Autodesk Inventor part; units mm, degrees
(part 2 of 4)
  line L489 (-4.322, 37.579) -> (-4.3544, 37.6135) construction
  line L490 (-4.3544, 37.6135) -> (-4.3855, 37.6466) construction
  line L491 (-4.3855, 37.6466) -> (-4.4003, 37.6527) construction
  line L492 (-4.4003, 37.6527) -> (-4.4094, 37.6363) construction
  line L493 (-4.4094, 37.6363) -> (-4.4207, 37.616) construction
  line L494 (-4.4207, 37.616) -> (-4.4319, 37.5271) construction
  line L495 (-4.4319, 37.5271) -> (-4.4272, 37.4953) construction
  line L496 (-4.4272, 37.4953) -> (-4.4241, 37.4748) construction
  line L497 (-4.4241, 37.4748) -> (-4.3492, 37.509) construction
  line L498 (-4.3492, 37.509) -> (-4.3297, 37.5398) construction
  spline S99 degree 3 poles (-4.2878, 37.7736) (-4.285, 37.7935) (-4.2987, 37.8243) (-4.3182, 37.842) (-4.353, 37.8735) (-4.3543, 37.8731) (-4.372, 37.8267) (-4.4023, 37.747) (-4.3954, 37.7255) (-4.3415, 37.7317) (-4.3084, 37.7355) (-4.2914, 37.7488) (-4.2878, 37.7736) knots 0 0 0 0 1 1 1 2 2 2 3 3 3 4 4 4 4
  line L499 (-4.2878, 37.7736) -> (-4.285, 37.7935) construction
  line L500 (-4.285, 37.7935) -> (-4.2987, 37.8243) construction
  line L501 (-4.2987, 37.8243) -> (-4.3182, 37.842) construction
  line L502 (-4.3182, 37.842) -> (-4.353, 37.8735) construction
  line L503 (-4.353, 37.8735) -> (-4.3543, 37.8731) construction
  line L504 (-4.3543, 37.8731) -> (-4.372, 37.8267) construction
  line L505 (-4.372, 37.8267) -> (-4.4023, 37.747) construction
  line L506 (-4.4023, 37.747) -> (-4.3954, 37.7255) construction
  line L507 (-4.3954, 37.7255) -> (-4.3415, 37.7317) construction
  line L508 (-4.3415, 37.7317) -> (-4.3084, 37.7355) construction
  line L509 (-4.3084, 37.7355) -> (-4.2914, 37.7488) construction
  line L510 (-4.2914, 37.7488) -> (-4.2878, 37.7736) construction
  spline S100 degree 3 poles (-4.2238, 37.9809) (-4.2021, 38.0154) (-4.229, 38.0724) (-4.267, 38.0724) (-4.3025, 38.0724) (-4.3297, 37.9751) (-4.2996, 37.956) (-4.2687, 37.9365) (-4.2474, 37.9435) (-4.2238, 37.9809) knots 0 0 0 0 1 1 1 2 2 2 3 3 3 3
  line L511 (-4.2238, 37.9809) -> (-4.2021, 38.0154) construction
  line L512 (-4.2021, 38.0154) -> (-4.229, 38.0724) construction
  line L513 (-4.229, 38.0724) -> (-4.267, 38.0724) construction
  line L514 (-4.267, 38.0724) -> (-4.3025, 38.0724) construction
  line L515 (-4.3025, 38.0724) -> (-4.3297, 37.9751) construction
  line L516 (-4.3297, 37.9751) -> (-4.2996, 37.956) construction
  line L517 (-4.2996, 37.956) -> (-4.2687, 37.9365) construction
  line L518 (-4.2687, 37.9365) -> (-4.2474, 37.9435) construction
  line L519 (-4.2474, 37.9435) -> (-4.2238, 37.9809) construction
  spline S101 degree 3 poles (-4.1426, 38.1788) (-4.1247, 38.2004) (-4.1246, 38.2154) (-4.1421, 38.2537) knots 0 0 0 0 1 1 1 1
  line L520 (-4.1426, 38.1788) -> (-4.1247, 38.2004) construction
  line L521 (-4.1247, 38.2004) -> (-4.1246, 38.2154) construction
  line L522 (-4.1246, 38.2154) -> (-4.1421, 38.2537) construction
  line L523 (-4.1421, 38.2537) -> (-4.1639, 38.3016)
  line L524 (-4.1639, 38.3016) -> (-4.1976, 38.26)
  spline S102 degree 3 poles (-4.1976, 38.26) (-4.2413, 38.206) (-4.2416, 38.1518) (-4.1982, 38.1518) (-4.1799, 38.1518) (-4.155, 38.164) (-4.1426, 38.1788) knots 3 3 3 3 4 4 4 5 5 5 5
  line L525 (-4.1976, 38.26) -> (-4.2413, 38.206) construction
  line L526 (-4.2413, 38.206) -> (-4.2416, 38.1518) construction
  line L527 (-4.2416, 38.1518) -> (-4.1982, 38.1518) construction
  line L528 (-4.1982, 38.1518) -> (-4.1799, 38.1518) construction
  line L529 (-4.1799, 38.1518) -> (-4.155, 38.164) construction
  line L530 (-4.155, 38.164) -> (-4.1426, 38.1788) construction
  spline S103 degree 3 poles (-4.038, 38.3715) (-4.0155, 38.3985) (-4.0284, 38.4693) (-4.0557, 38.4693) (-4.0805, 38.4693) (-4.1299, 38.3849) (-4.1171, 38.3643) (-4.1009, 38.338) (-4.0628, 38.3415) (-4.038, 38.3715) knots 0 0 0 0 1 1 1 2 2 2 3 3 3 3
  line L531 (-4.038, 38.3715) -> (-4.0155, 38.3985) construction
  line L532 (-4.0155, 38.3985) -> (-4.0284, 38.4693) construction
  line L533 (-4.0284, 38.4693) -> (-4.0557, 38.4693) construction
  line L534 (-4.0557, 38.4693) -> (-4.0805, 38.4693) construction
  line L535 (-4.0805, 38.4693) -> (-4.1299, 38.3849) construction
  line L536 (-4.1299, 38.3849) -> (-4.1171, 38.3643) construction
  line L537 (-4.1171, 38.3643) -> (-4.1009, 38.338) construction
  line L538 (-4.1009, 38.338) -> (-4.0628, 38.3415) construction
  line L539 (-4.0628, 38.3415) -> (-4.038, 38.3715) construction
  spline S104 degree 3 poles (-3.8872, 38.5577) (-3.8725, 38.5815) (-3.8939, 38.6457) (-3.9165, 38.6457) (-3.9358, 38.6457) (-4.0004, 38.5752) (-4.0014, 38.5531) knots 0 0 0 0 1 1 1 2 2 2 2
  line L540 (-3.8872, 38.5577) -> (-3.8725, 38.5815) construction
  line L541 (-3.8725, 38.5815) -> (-3.8939, 38.6457) construction
  line L542 (-3.8939, 38.6457) -> (-3.9165, 38.6457) construction
  line L543 (-3.9165, 38.6457) -> (-3.9358, 38.6457) construction
  line L544 (-3.9358, 38.6457) -> (-4.0004, 38.5752) construction
  line L545 (-4.0004, 38.5752) -> (-4.0014, 38.5531) construction
  spline S105 degree 3 poles (-4.0014, 38.5531) (-4.0023, 38.5331) (-3.8999, 38.5372) (-3.8872, 38.5577) knots 2 2 2 2 3 3 3 3
  line L546 (-4.0014, 38.5531) -> (-4.0023, 38.5331) construction
  line L547 (-4.0023, 38.5331) -> (-3.8999, 38.5372) construction
  line L548 (-3.8999, 38.5372) -> (-3.8872, 38.5577) construction
  spline S106 degree 3 poles (-3.7405, 38.7393) (-3.7371, 38.7569) (-3.7393, 38.7839) (-3.7452, 38.7995) knots 0 0 0 0 1 1 1 1
  line L549 (-3.7405, 38.7393) -> (-3.7371, 38.7569) construction
  line L550 (-3.7371, 38.7569) -> (-3.7393, 38.7839) construction
  line L551 (-3.7393, 38.7839) -> (-3.7452, 38.7995) construction
  spline S107 degree 3 poles (-3.7452, 38.7995) (-3.7543, 38.8232) (-3.7644, 38.8197) (-3.8078, 38.7781) knots 1 1 1 1 2 2 2 2
  line L552 (-3.7452, 38.7995) -> (-3.7543, 38.8232) construction
  line L553 (-3.7543, 38.8232) -> (-3.7644, 38.8197) construction
  line L554 (-3.7644, 38.8197) -> (-3.8078, 38.7781) construction
  spline S108 degree 3 poles (-3.8078, 38.7781) (-3.8363, 38.7508) (-3.8552, 38.7213) (-3.8497, 38.7126) knots 2 2 2 2 3 3 3 3
  line L555 (-3.8078, 38.7781) -> (-3.8363, 38.7508) construction
  line L556 (-3.8363, 38.7508) -> (-3.8552, 38.7213) construction
  line L557 (-3.8552, 38.7213) -> (-3.8497, 38.7126) construction
  spline S109 degree 3 poles (-3.8497, 38.7126) (-3.8323, 38.6844) (-3.7469, 38.7053) (-3.7405, 38.7393) knots 3 3 3 3 4 4 4 4
  line L558 (-3.8497, 38.7126) -> (-3.8323, 38.6844) construction
  line L559 (-3.8323, 38.6844) -> (-3.7469, 38.7053) construction
  line L560 (-3.7469, 38.7053) -> (-3.7405, 38.7393) construction
  spline S110 degree 3 poles (-3.5972, 38.8708) (-3.5719, 38.8912) (-3.5629, 38.9122) (-3.5706, 38.9325) (-3.5861, 38.9727) (-3.595, 38.9713) (-3.658, 38.9194) (-3.7025, 38.8828) (-3.7067, 38.873) (-3.6845, 38.8581) (-3.6486, 38.8339) (-3.6414, 38.835) (-3.5972, 38.8708) knots 0 0 0 0 1 1 1 2 2 2 3 3 3 4 4 4 4
  line L561 (-3.5972, 38.8708) -> (-3.5719, 38.8912) construction
  line L562 (-3.5719, 38.8912) -> (-3.5629, 38.9122) construction
  line L563 (-3.5629, 38.9122) -> (-3.5706, 38.9325) construction
  line L564 (-3.5706, 38.9325) -> (-3.5861, 38.9727) construction
  line L565 (-3.5861, 38.9727) -> (-3.595, 38.9713) construction
  line L566 (-3.595, 38.9713) -> (-3.658, 38.9194) construction
  line L567 (-3.658, 38.9194) -> (-3.7025, 38.8828) construction
  line L568 (-3.7025, 38.8828) -> (-3.7067, 38.873) construction
  line L569 (-3.7067, 38.873) -> (-3.6845, 38.8581) construction
  line L570 (-3.6845, 38.8581) -> (-3.6486, 38.8339) construction
  line L571 (-3.6486, 38.8339) -> (-3.6414, 38.835) construction
  line L572 (-3.6414, 38.835) -> (-3.5972, 38.8708) construction
  spline S111 degree 3 poles (-3.4055, 39.0382) (-3.399, 39.095) (-3.4114, 39.0978) (-3.477, 39.0546) (-3.5151, 39.0295) (-3.5208, 39.0182) (-3.5037, 39.0011) (-3.4664, 38.9638) (-3.4117, 38.9845) (-3.4055, 39.0382) knots 0 0 0 0 1 1 1 2 2 2 3 3 3 3
  line L573 (-3.4055, 39.0382) -> (-3.399, 39.095) construction
  line L574 (-3.399, 39.095) -> (-3.4114, 39.0978) construction
  line L575 (-3.4114, 39.0978) -> (-3.477, 39.0546) construction
  line L576 (-3.477, 39.0546) -> (-3.5151, 39.0295) construction
  line L577 (-3.5151, 39.0295) -> (-3.5208, 39.0182) construction
  line L578 (-3.5208, 39.0182) -> (-3.5037, 39.0011) construction
  line L579 (-3.5037, 39.0011) -> (-3.4664, 38.9638) construction
  line L580 (-3.4664, 38.9638) -> (-3.4117, 38.9845) construction
  line L581 (-3.4117, 38.9845) -> (-3.4055, 39.0382) construction
  spline S112 degree 3 poles (-1.0519, 39.023) (-1.0061, 39.0578) (-1.0139, 39.0747) (-1.0906, 39.1069) (-1.1666, 39.1388) (-1.1798, 39.1346) (-1.1798, 39.0784) (-1.1798, 39.0055) (-1.113, 38.9766) (-1.0519, 39.023) knots 0 0 0 0 1 1 1 2 2 2 3 3 3 3
  line L582 (-1.0519, 39.023) -> (-1.0061, 39.0578) construction
  line L583 (-1.0061, 39.0578) -> (-1.0139, 39.0747) construction
  line L584 (-1.0139, 39.0747) -> (-1.0906, 39.1069) construction
  line L585 (-1.0906, 39.1069) -> (-1.1666, 39.1388) construction
  line L586 (-1.1666, 39.1388) -> (-1.1798, 39.1346) construction
  line L587 (-1.1798, 39.1346) -> (-1.1798, 39.0784) construction
  line L588 (-1.1798, 39.0784) -> (-1.1798, 39.0055) construction
  line L589 (-1.1798, 39.0055) -> (-1.113, 38.9766) construction
  line L590 (-1.113, 38.9766) -> (-1.0519, 39.023) construction
  spline S113 degree 3 poles (-3.2361, 39.0974) (-3.2196, 39.1037) (-3.2082, 39.1288) (-3.2082, 39.1588) knots 0 0 0 0 1 1 1 1
  line L591 (-3.2361, 39.0974) -> (-3.2196, 39.1037) construction
  line L592 (-3.2196, 39.1037) -> (-3.2082, 39.1288) construction
  line L593 (-3.2082, 39.1288) -> (-3.2082, 39.1588) construction
  line L594 (-3.2082, 39.1588) -> (-3.2082, 39.2096)
  line L595 (-3.2082, 39.2096) -> (-3.27, 39.1801)
  spline S114 degree 3 poles (-3.27, 39.1801) (-3.3393, 39.1471) (-3.3456, 39.1318) (-3.3008, 39.1057) knots 3 3 3 3 4 4 4 4
  line L596 (-3.27, 39.1801) -> (-3.3393, 39.1471) construction
  line L597 (-3.3393, 39.1471) -> (-3.3456, 39.1318) construction
  line L598 (-3.3456, 39.1318) -> (-3.3008, 39.1057) construction
  spline S115 degree 3 poles (-3.3008, 39.1057) (-3.2631, 39.0838) (-3.2695, 39.0846) (-3.2361, 39.0974) knots 4 4 4 4 5 5 5 5
  line L599 (-3.3008, 39.1057) -> (-3.2631, 39.0838) construction
  line L600 (-3.2631, 39.0838) -> (-3.2695, 39.0846) construction
  line L601 (-3.2695, 39.0846) -> (-3.2361, 39.0974) construction
  spline S116 degree 3 poles (-1.2604, 39.1312) (-1.2417, 39.1453) (-1.2298, 39.1599) (-1.234, 39.1636) knots 0 0 0 0 1 1 1 1
  line L602 (-1.2604, 39.1312) -> (-1.2417, 39.1453) construction
  line L603 (-1.2417, 39.1453) -> (-1.2298, 39.1599) construction
  line L604 (-1.2298, 39.1599) -> (-1.234, 39.1636) construction
  spline S117 degree 3 poles (-1.234, 39.1636) (-1.2466, 39.175) (-1.3537, 39.2278) (-1.3641, 39.2278) (-1.3827, 39.2278) (-1.3736, 39.1465) (-1.3526, 39.1255) (-1.3252, 39.0981) (-1.3023, 39.0995) (-1.2604, 39.1312) knots 1 1 1 1 2 2 2 3 3 3 4 4 4 4
  line L605 (-1.234, 39.1636) -> (-1.2466, 39.175) construction
  line L606 (-1.2466, 39.175) -> (-1.3537, 39.2278) construction
  line L607 (-1.3537, 39.2278) -> (-1.3641, 39.2278) construction
  line L608 (-1.3641, 39.2278) -> (-1.3827, 39.2278) construction
  line L609 (-1.3827, 39.2278) -> (-1.3736, 39.1465) construction
  line L610 (-1.3736, 39.1465) -> (-1.3526, 39.1255) construction
  line L611 (-1.3526, 39.1255) -> (-1.3252, 39.0981) construction
  line L612 (-1.3252, 39.0981) -> (-1.3023, 39.0995) construction
  line L613 (-1.3023, 39.0995) -> (-1.2604, 39.1312) construction
  spline S118 degree 3 poles (-3.0073, 39.2204) (-2.9897, 39.2662) (-2.9948, 39.2807) (-3.0285, 39.2807) (-3.0735, 39.2807) (-3.1278, 39.237) (-3.1129, 39.2128) (-3.0943, 39.1828) (-3.0196, 39.1882) (-3.0073, 39.2204) knots 0 0 0 0 1 1 1 2 2 2 3 3 3 3
  line L614 (-3.0073, 39.2204) -> (-2.9897, 39.2662) construction
  line L615 (-2.9897, 39.2662) -> (-2.9948, 39.2807) construction
  line L616 (-2.9948, 39.2807) -> (-3.0285, 39.2807) construction
  line L617 (-3.0285, 39.2807) -> (-3.0735, 39.2807) construction
  line L618 (-3.0735, 39.2807) -> (-3.1278, 39.237) construction
  line L619 (-3.1278, 39.237) -> (-3.1129, 39.2128) construction
  line L620 (-3.1129, 39.2128) -> (-3.0943, 39.1828) construction
  line L621 (-3.0943, 39.1828) -> (-3.0196, 39.1882) construction
  line L622 (-3.0196, 39.1882) -> (-3.0073, 39.2204) construction
  spline S119 degree 3 poles (-1.4709, 39.2214) (-1.4551, 39.2372) (-1.4485, 39.2556) (-1.4564, 39.2621) (-1.4852, 39.2859) (-1.5646, 39.3133) (-1.5749, 39.303) (-1.5962, 39.2817) (-1.5846, 39.229) (-1.5546, 39.2116) (-1.5126, 39.1871) (-1.5042, 39.1881) (-1.4709, 39.2214) knots 0 0 0 0 1 1 1 2 2 2 3 3 3 4 4 4 4
  line L623 (-1.4709, 39.2214) -> (-1.4551, 39.2372) construction
  line L624 (-1.4551, 39.2372) -> (-1.4485, 39.2556) construction
  line L625 (-1.4485, 39.2556) -> (-1.4564, 39.2621) construction
  line L626 (-1.4564, 39.2621) -> (-1.4852, 39.2859) construction
  line L627 (-1.4852, 39.2859) -> (-1.5646, 39.3133) construction
  line L628 (-1.5646, 39.3133) -> (-1.5749, 39.303) construction
  line L629 (-1.5749, 39.303) -> (-1.5962, 39.2817) construction
  line L630 (-1.5962, 39.2817) -> (-1.5846, 39.229) construction
  line L631 (-1.5846, 39.229) -> (-1.5546, 39.2116) construction
  line L632 (-1.5546, 39.2116) -> (-1.5126, 39.1871) construction
  line L633 (-1.5126, 39.1871) -> (-1.5042, 39.1881) construction
  line L634 (-1.5042, 39.1881) -> (-1.4709, 39.2214) construction
  spline S120 degree 3 poles (-2.7877, 39.3141) (-2.7822, 39.3531) (-2.7862, 39.3554) (-2.8394, 39.3448) (-2.9095, 39.3307) (-2.9157, 39.3252) (-2.9018, 39.2891) (-2.884, 39.2428) (-2.7951, 39.2622) (-2.7877, 39.3141) knots 0 0 0 0 1 1 1 2 2 2 3 3 3 3
  line L635 (-2.7877, 39.3141) -> (-2.7822, 39.3531) construction
  line L636 (-2.7822, 39.3531) -> (-2.7862, 39.3554) construction
  line L637 (-2.7862, 39.3554) -> (-2.8394, 39.3448) construction
  line L638 (-2.8394, 39.3448) -> (-2.9095, 39.3307) construction
  line L639 (-2.9095, 39.3307) -> (-2.9157, 39.3252) construction
  line L640 (-2.9157, 39.3252) -> (-2.9018, 39.2891) construction
  line L641 (-2.9018, 39.2891) -> (-2.884, 39.2428) construction
  line L642 (-2.884, 39.2428) -> (-2.7951, 39.2622) construction
  line L643 (-2.7951, 39.2622) -> (-2.7877, 39.3141) construction
  spline S121 degree 3 poles (-1.6647, 39.3161) (-1.6529, 39.3353) (-1.7263, 39.3689) (-1.7801, 39.3689) (-1.8184, 39.3689) (-1.8103, 39.3218) (-1.7658, 39.2858) (-1.7387, 39.2639) (-1.6875, 39.2793) (-1.6647, 39.3161) knots 0 0 0 0 1 1 1 2 2 2 3 3 3 3
  line L644 (-1.6647, 39.3161) -> (-1.6529, 39.3353) construction
  line L645 (-1.6529, 39.3353) -> (-1.7263, 39.3689) construction
  line L646 (-1.7263, 39.3689) -> (-1.7801, 39.3689) construction
  line L647 (-1.7801, 39.3689) -> (-1.8184, 39.3689) construction
  line L648 (-1.8184, 39.3689) -> (-1.8103, 39.3218) construction
  line L649 (-1.8103, 39.3218) -> (-1.7658, 39.2858) construction
  line L650 (-1.7658, 39.2858) -> (-1.7387, 39.2639) construction
  line L651 (-1.7387, 39.2639) -> (-1.6875, 39.2793) construction
  line L652 (-1.6875, 39.2793) -> (-1.6647, 39.3161) construction
  spline S122 degree 3 poles (-2.5767, 39.3372) (-2.5324, 39.3815) (-2.5521, 39.4064) (-2.6217, 39.3938) knots 0 0 0 0 1 1 1 1
  line L653 (-2.5767, 39.3372) -> (-2.5324, 39.3815) construction
  line L654 (-2.5324, 39.3815) -> (-2.5521, 39.4064) construction
  line L655 (-2.5521, 39.4064) -> (-2.6217, 39.3938) construction
  spline S123 degree 3 poles (-2.6217, 39.3938) (-2.7038, 39.379) (-2.707, 39.3761) (-2.6794, 39.3429) knots 1 1 1 1 2 2 2 2
  line L656 (-2.6217, 39.3938) -> (-2.7038, 39.379) construction
  line L657 (-2.7038, 39.379) -> (-2.707, 39.3761) construction
  line L658 (-2.707, 39.3761) -> (-2.6794, 39.3429) construction
  spline S124 degree 3 poles (-2.6794, 39.3429) (-2.6527, 39.3106) (-2.6059, 39.308) (-2.5767, 39.3372) knots 2 2 2 2 3 3 3 3
  line L659 (-2.6794, 39.3429) -> (-2.6527, 39.3106) construction
  line L660 (-2.6527, 39.3106) -> (-2.6059, 39.308) construction
  line L661 (-2.6059, 39.308) -> (-2.5767, 39.3372) construction
  spline S125 degree 3 poles (-1.9018, 39.3438) (-1.8827, 39.3668) (-1.8831, 39.3743) (-1.9041, 39.3876) (-1.9426, 39.412) (-2.0264, 39.4076) (-2.0264, 39.3812) (-2.0264, 39.3207) (-1.9421, 39.2953) (-1.9018, 39.3438) knots 0 0 0 0 1 1 1 2 2 2 3 3 3 3
  line L662 (-1.9018, 39.3438) -> (-1.8827, 39.3668) construction
  line L663 (-1.8827, 39.3668) -> (-1.8831, 39.3743) construction
  line L664 (-1.8831, 39.3743) -> (-1.9041, 39.3876) construction
  line L665 (-1.9041, 39.3876) -> (-1.9426, 39.412) construction
  line L666 (-1.9426, 39.412) -> (-2.0264, 39.4076) construction
  line L667 (-2.0264, 39.4076) -> (-2.0264, 39.3812) construction
  line L668 (-2.0264, 39.3812) -> (-2.0264, 39.3207) construction
  line L669 (-2.0264, 39.3207) -> (-1.9421, 39.2953) construction
  line L670 (-1.9421, 39.2953) -> (-1.9018, 39.3438) construction
  spline S126 degree 3 poles (-2.3445, 39.3678) (-2.3221, 39.4097) (-2.3393, 39.4222) (-2.407, 39.4133) knots 0 0 0 0 1 1 1 1
  line L671 (-2.3445, 39.3678) -> (-2.3221, 39.4097) construction
  line L672 (-2.3221, 39.4097) -> (-2.3393, 39.4222) construction
  line L673 (-2.3393, 39.4222) -> (-2.407, 39.4133) construction
  spline S127 degree 3 poles (-2.407, 39.4133) (-2.4354, 39.4096) (-2.4657, 39.4061) (-2.4745, 39.4054) knots 1 1 1 1 2 2 2 2
  line L674 (-2.407, 39.4133) -> (-2.4354, 39.4096) construction
  line L675 (-2.4354, 39.4096) -> (-2.4657, 39.4061) construction
  line L676 (-2.4657, 39.4061) -> (-2.4745, 39.4054) construction
  spline S128 degree 3 poles (-2.4745, 39.4054) (-2.5042, 39.4031) (-2.4269, 39.3336) (-2.3947, 39.3336) (-2.3772, 39.3336) (-2.3546, 39.349) (-2.3445, 39.3678) knots 2 2 2 2 3 3 3 4 4 4 4
  line L677 (-2.4745, 39.4054) -> (-2.5042, 39.4031) construction
  line L678 (-2.5042, 39.4031) -> (-2.4269, 39.3336) construction
  line L679 (-2.4269, 39.3336) -> (-2.3947, 39.3336) construction
  line L680 (-2.3947, 39.3336) -> (-2.3772, 39.3336) construction
  line L681 (-2.3772, 39.3336) -> (-2.3546, 39.349) construction
  line L682 (-2.3546, 39.349) -> (-2.3445, 39.3678) construction
  spline S129 degree 3 poles (-2.1234, 39.3758) (-2.1234, 39.399) (-2.138, 39.4106) (-2.1717, 39.4142) (-2.2288, 39.4203) (-2.2499, 39.3955) (-2.2191, 39.3585) (-2.1888, 39.322) (-2.1234, 39.3338) (-2.1234, 39.3758) knots 0 0 0 0 1 1 1 2 2 2 3 3 3 3
  line L683 (-2.1234, 39.3758) -> (-2.1234, 39.399) construction
  line L684 (-2.1234, 39.399) -> (-2.138, 39.4106) construction
  line L685 (-2.138, 39.4106) -> (-2.1717, 39.4142) construction
  line L686 (-2.1717, 39.4142) -> (-2.2288, 39.4203) construction
  line L687 (-2.2288, 39.4203) -> (-2.2499, 39.3955) construction
  line L688 (-2.2499, 39.3955) -> (-2.2191, 39.3585) construction
  line L689 (-2.2191, 39.3585) -> (-2.1888, 39.322) construction
  line L690 (-2.1888, 39.322) -> (-2.1234, 39.3338) construction
  line L691 (-2.1234, 39.3338) -> (-2.1234, 39.3758) construction
  spline S130 degree 3 poles (1.5366, 35.9381) (1.0352, 36.0392) (0.6343, 36.4249) (0.5246, 36.9118) knots 0 0 0 0 1 1 1 1
  line L692 (1.5366, 35.9381) -> (1.0352, 36.0392) construction
  line L693 (1.0352, 36.0392) -> (0.6343, 36.4249) construction
  line L694 (0.6343, 36.4249) -> (0.5246, 36.9118) construction
  spline S131 degree 3 poles (0.5246, 36.9118) (0.4888, 37.0703) (0.488, 37.3485) (0.5228, 37.4962) knots 1 1 1 1 2 2 2 2
  line L695 (0.5246, 36.9118) -> (0.4888, 37.0703) construction
  line L696 (0.4888, 37.0703) -> (0.488, 37.3485) construction
  line L697 (0.488, 37.3485) -> (0.5228, 37.4962) construction
  spline S132 degree 3 poles (0.5228, 37.4962) (0.6143, 37.8845) (0.9204, 38.2576) (1.1475, 38.2576) (1.1854, 38.2576) (1.26, 38.2264) (1.3611, 38.168) knots 2 2 2 2 3 3 3 4 4 4 4
  line L698 (0.5228, 37.4962) -> (0.6143, 37.8845) construction
  line L699 (0.6143, 37.8845) -> (0.9204, 38.2576) construction
  line L700 (0.9204, 38.2576) -> (1.1475, 38.2576) construction
  line L701 (1.1475, 38.2576) -> (1.1854, 38.2576) construction
  line L702 (1.1854, 38.2576) -> (1.26, 38.2264) construction
  line L703 (1.26, 38.2264) -> (1.3611, 38.168) construction
  spline S133 degree 3 poles (1.3611, 38.168) (1.5814, 38.0409) (1.6967, 38.0076) (1.9511, 37.9978) knots 4 4 4 4 5 5 5 5
  line L704 (1.3611, 38.168) -> (1.5814, 38.0409) construction
  line L705 (1.5814, 38.0409) -> (1.6967, 38.0076) construction
  line L706 (1.6967, 38.0076) -> (1.9511, 37.9978) construction
  spline S134 degree 3 poles (1.9511, 37.9978) (2.1285, 37.9909) (2.1996, 37.9968) (2.3898, 38.0341) knots 5 5 5 5 6 6 6 6
  line L707 (1.9511, 37.9978) -> (2.1285, 37.9909) construction
  line L708 (2.1285, 37.9909) -> (2.1996, 37.9968) construction
  line L709 (2.1996, 37.9968) -> (2.3898, 38.0341) construction
  spline S135 degree 3 poles (2.3898, 38.0341) (2.5146, 38.0586) (2.6297, 38.074) (2.6455, 38.0685) knots 6 6 6 6 7 7 7 7
  line L710 (2.3898, 38.0341) -> (2.5146, 38.0586) construction
  line L711 (2.5146, 38.0586) -> (2.6297, 38.074) construction
  line L712 (2.6297, 38.074) -> (2.6455, 38.0685) construction
  spline S136 degree 3 poles (2.6455, 38.0685) (2.8039, 38.0131) (2.9769, 37.719) (2.9313, 37.583) knots 7 7 7 7 8 8 8 8
  line L713 (2.6455, 38.0685) -> (2.8039, 38.0131) construction
  line L714 (2.8039, 38.0131) -> (2.9769, 37.719) construction
  line L715 (2.9769, 37.719) -> (2.9313, 37.583) construction
  spline S137 degree 3 poles (2.9313, 37.583) (2.9207, 37.5515) (2.8523, 37.4502) (2.7793, 37.3581) knots 8 8 8 8 9 9 9 9
  line L716 (2.9313, 37.583) -> (2.9207, 37.5515) construction
  line L717 (2.9207, 37.5515) -> (2.8523, 37.4502) construction
  line L718 (2.8523, 37.4502) -> (2.7793, 37.3581) construction
  spline S138 degree 3 poles (2.7793, 37.3581) (2.6299, 37.1693) (2.5212, 36.9634) (2.4813, 36.7936) knots 9 9 9 9 10 10 10 10
  line L719 (2.7793, 37.3581) -> (2.6299, 37.1693) construction
  line L720 (2.6299, 37.1693) -> (2.5212, 36.9634) construction
  line L721 (2.5212, 36.9634) -> (2.4813, 36.7936) construction
  spline S139 degree 3 poles (2.4813, 36.7936) (2.4637, 36.7188) (2.4543, 36.5898) (2.4541, 36.4224) knots 10 10 10 10 11 11 11 11
  line L722 (2.4813, 36.7936) -> (2.4637, 36.7188) construction
  line L723 (2.4637, 36.7188) -> (2.4543, 36.5898) construction
  line L724 (2.4543, 36.5898) -> (2.4541, 36.4224) construction
  line L725 (2.4541, 36.4224) -> (2.4539, 36.1658)
  line L726 (2.4539, 36.1658) -> (2.3877, 36.1015)
  spline S140 degree 3 poles (2.3877, 36.1015) (2.2294, 35.9478) (1.85, 35.8749) (1.5366, 35.9381) knots 13 13 13 13 14 14 14 14
  line L727 (2.3877, 36.1015) -> (2.2294, 35.9478) construction
  line L728 (2.2294, 35.9478) -> (1.85, 35.8749) construction
  line L729 (1.85, 35.8749) -> (1.5366, 35.9381) construction
  line L730 (1.5366, 35.9381) -> (1.5366, 35.9381)
  spline S141 degree 3 poles (1.9223, 37.0184) (2.0275, 37.0968) (2.0617, 37.2291) (2.005, 37.3387) (1.8856, 37.5695) (1.5194, 37.4556) (1.5419, 37.1947) (1.5496, 37.1055) (1.5809, 37.0579) (1.6689, 37.0018) (1.7345, 36.96) (1.8545, 36.9679) (1.9223, 37.0184) knots 0 0 0 0 1 1 1 2 2 2 3 3 3 4 4 4 4
  line L731 (1.9223, 37.0184) -> (2.0275, 37.0968) construction
  line L732 (2.0275, 37.0968) -> (2.0617, 37.2291) construction
  line L733 (2.0617, 37.2291) -> (2.005, 37.3387) construction
  line L734 (2.005, 37.3387) -> (1.8856, 37.5695) construction
  line L735 (1.8856, 37.5695) -> (1.5194, 37.4556) construction
  line L736 (1.5194, 37.4556) -> (1.5419, 37.1947) construction
  line L737 (1.5419, 37.1947) -> (1.5496, 37.1055) construction
  line L738 (1.5496, 37.1055) -> (1.5809, 37.0579) construction
  line L739 (1.5809, 37.0579) -> (1.6689, 37.0018) construction
  line L740 (1.6689, 37.0018) -> (1.7345, 36.96) construction
  line L741 (1.7345, 36.96) -> (1.8545, 36.9679) construction
  line L742 (1.8545, 36.9679) -> (1.9223, 37.0184) construction
  spline S142 degree 3 poles (2.7347, 37.633) (2.7738, 37.6659) (2.789, 37.694) (2.789, 37.7333) (2.789, 37.884) (2.5831, 37.9231) (2.5252, 37.7834) knots 0 0 0 0 1 1 1 2 2 2 2
  line L743 (2.7347, 37.633) -> (2.7738, 37.6659) construction
  line L744 (2.7738, 37.6659) -> (2.789, 37.694) construction
  line L745 (2.789, 37.694) -> (2.789, 37.7333) construction
  line L746 (2.789, 37.7333) -> (2.789, 37.884) construction
  line L747 (2.789, 37.884) -> (2.5831, 37.9231) construction
  line L748 (2.5831, 37.9231) -> (2.5252, 37.7834) construction
  spline S143 degree 3 poles (2.5252, 37.7834) (2.4983, 37.7185) (2.5284, 37.6439) (2.595, 37.6102) knots 2 2 2 2 3 3 3 3
  line L749 (2.5252, 37.7834) -> (2.4983, 37.7185) construction
  line L750 (2.4983, 37.7185) -> (2.5284, 37.6439) construction
  line L751 (2.5284, 37.6439) -> (2.595, 37.6102) construction
  spline S144 degree 3 poles (2.595, 37.6102) (2.6571, 37.5788) (2.6734, 37.5814) (2.7347, 37.633) knots 3 3 3 3 4 4 4 4
  line L752 (2.595, 37.6102) -> (2.6571, 37.5788) construction
  line L753 (2.6571, 37.5788) -> (2.6734, 37.5814) construction
  line L754 (2.6734, 37.5814) -> (2.7347, 37.633) construction
  spline S145 degree 3 poles (2.24, 38.1915) (2.2243, 38.2425) (2.095, 38.6453) (1.9528, 39.0867) (1.8106, 39.5281) (1.662, 39.9983) (1.6227, 40.1315) knots 0 0 0 0 1 1 1 2 2 2 2
  line L755 (2.24, 38.1915) -> (2.2243, 38.2425) construction
  line L756 (2.2243, 38.2425) -> (2.095, 38.6453) construction
  line L757 (2.095, 38.6453) -> (1.9528, 39.0867) construction
  line L758 (1.9528, 39.0867) -> (1.8106, 39.5281) construction
  line L759 (1.8106, 39.5281) -> (1.662, 39.9983) construction
  line L760 (1.662, 39.9983) -> (1.6227, 40.1315) construction
  line L761 (1.6227, 40.1315) -> (1.5511, 40.3738)
  line L762 (1.5511, 40.3738) -> (1.5836, 40.44)
  spline S146 degree 3 poles (1.5836, 40.44) (1.6205, 40.5153) (1.7152, 40.586) (1.7791, 40.586) (1.8396, 40.586) (1.9294, 40.5402) (1.9576, 40.4951) knots 4 4 4 4 5 5 5 6 6 6 6
  line L763 (1.5836, 40.44) -> (1.6205, 40.5153) construction
  line L764 (1.6205, 40.5153) -> (1.7152, 40.586) construction
  line L765 (1.7152, 40.586) -> (1.7791, 40.586) construction
  line L766 (1.7791, 40.586) -> (1.8396, 40.586) construction
  line L767 (1.8396, 40.586) -> (1.9294, 40.5402) construction
  line L768 (1.9294, 40.5402) -> (1.9576, 40.4951) construction
  spline S147 degree 3 poles (1.9576, 40.4951) (1.9706, 40.4742) (2.1109, 40.0753) (2.2693, 39.6087) knots 6 6 6 6 7 7 7 7
  line L769 (1.9576, 40.4951) -> (1.9706, 40.4742) construction
  line L770 (1.9706, 40.4742) -> (2.1109, 40.0753) construction
  line L771 (2.1109, 40.0753) -> (2.2693, 39.6087) construction
  spline S148 degree 3 poles (2.2693, 39.6087) (2.4278, 39.1421) (2.5734, 38.7167) (2.593, 38.6633) knots 7 7 7 7 8 8 8 8
  line L772 (2.2693, 39.6087) -> (2.4278, 39.1421) construction
  line L773 (2.4278, 39.1421) -> (2.5734, 38.7167) construction
  line L774 (2.5734, 38.7167) -> (2.593, 38.6633) construction
  spline S149 degree 3 poles (2.593, 38.6633) (2.6413, 38.5317) (2.7681, 38.1265) (2.7628, 38.1204) knots 8 8 8 8 9 9 9 9
  line L775 (2.593, 38.6633) -> (2.6413, 38.5317) construction
  line L776 (2.6413, 38.5317) -> (2.7681, 38.1265) construction
  line L777 (2.7681, 38.1265) -> (2.7628, 38.1204) construction
  spline S150 degree 3 poles (2.7628, 38.1204) (2.7605, 38.1178) (2.7371, 38.1237) (2.7109, 38.1337) knots 9 9 9 9 10 10 10 10
  line L778 (2.7628, 38.1204) -> (2.7605, 38.1178) construction
  line L779 (2.7605, 38.1178) -> (2.7371, 38.1237) construction
  line L780 (2.7371, 38.1237) -> (2.7109, 38.1337) construction
  spline S151 degree 3 poles (2.7109, 38.1337) (2.6441, 38.1591) (2.5324, 38.1559) (2.4186, 38.1254) knots 10 10 10 10 11 11 11 11
  line L781 (2.7109, 38.1337) -> (2.6441, 38.1591) construction
  line L782 (2.6441, 38.1591) -> (2.5324, 38.1559) construction
  line L783 (2.5324, 38.1559) -> (2.4186, 38.1254) construction
  spline S152 degree 3 poles (2.4186, 38.1254) (2.2755, 38.0869) (2.272, 38.0883) (2.24, 38.1915) knots 11 11 11 11 12 12 12 12
  line L784 (2.4186, 38.1254) -> (2.2755, 38.0869) construction
  line L785 (2.2755, 38.0869) -> (2.272, 38.0883) construction
  line L786 (2.272, 38.0883) -> (2.24, 38.1915) construction
  spline S153 degree 3 poles (1.8624, 40.2679) (1.9597, 40.3753) (1.8049, 40.5389) (1.701, 40.4386) (1.6588, 40.3978) (1.6565, 40.3307) (1.6957, 40.281) (1.741, 40.2234) (1.8168, 40.2174) (1.8624, 40.2679) knots 0 0 0 0 1 1 1 2 2 2 3 3 3 3
  line L787 (1.8624, 40.2679) -> (1.9597, 40.3753) construction
  line L788 (1.9597, 40.3753) -> (1.8049, 40.5389) construction
  line L789 (1.8049, 40.5389) -> (1.701, 40.4386) construction
  line L790 (1.701, 40.4386) -> (1.6588, 40.3978) construction
  line L791 (1.6588, 40.3978) -> (1.6565, 40.3307) construction
  line L792 (1.6565, 40.3307) -> (1.6957, 40.281) construction
  line L793 (1.6957, 40.281) -> (1.741, 40.2234) construction
  line L794 (1.741, 40.2234) -> (1.8168, 40.2174) construction
  line L795 (1.8168, 40.2174) -> (1.8624, 40.2679) construction
  spline S154 degree 3 poles (-3.6977, 39.9094) (-3.715, 39.9167) (-3.7198, 40.1679) (-3.7198, 41.0811) knots 0 0 0 0 1 1 1 1
  line L796 (-3.6977, 39.9094) -> (-3.715, 39.9167) construction
  line L797 (-3.715, 39.9167) -> (-3.7198, 40.1679) construction
  line L798 (-3.7198, 40.1679) -> (-3.7198, 41.0811) construction
  line L799 (-3.7198, 41.0811) -> (-3.7198, 42.2436)
  line L800 (-3.7198, 42.2436) -> (-4.3239, 42.2482)
  line L801 (-4.3239, 42.2482) -> (-4.928, 42.2529)
  line L802 (-4.928, 42.2529) -> (-4.928, 42.3058)
  line L803 (-4.928, 42.3058) -> (-4.928, 42.3587)
  line L804 (-4.928, 42.3587) -> (-3.6492, 42.3587)
  line L805 (-3.6492, 42.3587) -> (-2.3704, 42.3587)
  line L806 (-2.3704, 42.3587) -> (-2.3704, 42.3005)
  line L807 (-2.3704, 42.3005) -> (-2.3704, 42.2422)
  line L808 (-2.3704, 42.2422) -> (-2.9744, 42.2436)
  line L809 (-2.9744, 42.2436) -> (-3.5784, 42.2449)
  line L810 (-3.5784, 42.2449) -> (-3.5829, 41.0759)
  line L811 (-3.5829, 41.0759) -> (-3.5875, 39.9069)
  line L812 (-3.5875, 39.9069) -> (-3.6316, 39.9035)
  spline S155 degree 3 poles (-3.6316, 39.9035) (-3.6558, 39.9016) (-3.6856, 39.9042) (-3.6977, 39.9094) knots 15 15 15 15 16 16 16 16
  line L813 (-3.6316, 39.9035) -> (-3.6558, 39.9016) construction
  line L814 (-3.6558, 39.9016) -> (-3.6856, 39.9042) construction
  line L815 (-3.6856, 39.9042) -> (-3.6977, 39.9094) construction
  spline S156 degree 3 poles (-2.2123, 39.92) (-2.217, 39.9322) (-2.2187, 40.4859) (-2.2162, 41.1504) knots 0 0 0 0 1 1 1 1
  line L816 (-2.2123, 39.92) -> (-2.217, 39.9322) construction
  line L817 (-2.217, 39.9322) -> (-2.2187, 40.4859) construction
  line L818 (-2.2187, 40.4859) -> (-2.2162, 41.1504) construction
  line L819 (-2.2162, 41.1504) -> (-2.2116, 42.3587)
  line L820 (-2.2116, 42.3587) -> (-0.9284, 42.3632)
  line L821 (-0.9284, 42.3632) -> (0.3548, 42.3677)
  line L822 (0.3548, 42.3677) -> (0.3548, 42.3059)
  line L823 (0.3548, 42.3059) -> (0.3548, 42.244)
  line L824 (0.3548, 42.244) -> (-0.8711, 42.244)
  line L825 (-0.8711, 42.244) -> (-2.097, 42.244)
  line L826 (-2.097, 42.244) -> (-2.097, 41.7237)
  line L827 (-2.097, 41.7237) -> (-2.097, 41.2033)
  line L828 (-2.097, 41.2033) -> (-0.87, 41.2033)
  line L829 (-0.87, 41.2033) -> (0.357, 41.2033)
  line L830 (0.357, 41.2033) -> (0.3515, 41.1372)
  line L831 (0.3515, 41.1372) -> (0.346, 41.0711)
  line L832 (0.346, 41.0711) -> (-0.8755, 41.0665)
  line L833 (-0.8755, 41.0665) -> (-2.097, 41.062)
  line L834 (-2.097, 41.062) -> (-2.097, 40.5507)
  line L835 (-2.097, 40.5507) -> (-2.097, 40.0394)
  line L836 (-2.097, 40.0394) -> (-0.8755, 40.0349)
  line L837 (-0.8755, 40.0349) -> (0.346, 40.0304)
  line L838 (0.346, 40.0304) -> (0.346, 39.9686)
  line L839 (0.346, 39.9686) -> (0.346, 39.9069)
  line L840 (0.346, 39.9069) -> (-0.9289, 39.9024)
  spline S157 degree 3 poles (-0.9289, 39.9024) (-1.9395, 39.8988) (-2.2056, 39.9024) (-2.2123, 39.92) knots 23 23 23 23 24 24 24 24
  line L841 (-0.9289, 39.9024) -> (-1.9395, 39.8988) construction
  line L842 (-1.9395, 39.8988) -> (-2.2056, 39.9024) construction
  line L843 (-2.2056, 39.9024) -> (-2.2123, 39.92) construction
  spline S158 degree 3 poles (0.5045, 39.9189) (0.4996, 39.9317) (0.4977, 40.4859) (0.5002, 41.1504) knots 0 0 0 0 1 1 1 1
  line L844 (0.5045, 39.9189) -> (0.4996, 39.9317) construction
  line L845 (0.4996, 39.9317) -> (0.4977, 40.4859) construction
  line L846 (0.4977, 40.4859) -> (0.5002, 41.1504) construction
  line L847 (0.5002, 41.1504) -> (0.5048, 42.3587)
  line L848 (0.5048, 42.3587) -> (1.7836, 42.3587)
  line L849 (1.7836, 42.3587) -> (3.0624, 42.3587)
  line L850 (3.0624, 42.3587) -> (3.0624, 41.1328)
  line L851 (3.0624, 41.1328) -> (3.0624, 39.9069)
  line L852 (3.0624, 39.9069) -> (3.0207, 39.901)
  spline S159 degree 3 poles (3.0207, 39.901) (2.9977, 39.8977) (2.972, 39.902) (2.9635, 39.9105) knots 7 7 7 7 8 8 8 8
  line L853 (3.0207, 39.901) -> (2.9977, 39.8977) construction
  line L854 (2.9977, 39.8977) -> (2.972, 39.902) construction
  line L855 (2.972, 39.902) -> (2.9635, 39.9105) construction
  spline S160 degree 3 poles (2.9635, 39.9105) (2.955, 39.919) (2.947, 40.4476) (2.9458, 41.085) knots 8 8 8 8 9 9 9 9
  line L856 (2.9635, 39.9105) -> (2.955, 39.919) construction
  line L857 (2.955, 39.919) -> (2.947, 40.4476) construction
  line L858 (2.947, 40.4476) -> (2.9458, 41.085) construction
  line L859 (2.9458, 41.085) -> (2.9436, 42.244)
  line L860 (2.9436, 42.244) -> (1.7817, 42.244)
  line L861 (1.7817, 42.244) -> (0.6197, 42.244)
  line L862 (0.6197, 42.244) -> (0.6151, 41.0755)
  line L863 (0.6151, 41.0755) -> (0.6106, 39.9069)
  line L864 (0.6106, 39.9069) -> (0.562, 39.9013)
  spline S161 degree 3 poles (0.562, 39.9013) (0.5336, 39.898) (0.5097, 39.9054) (0.5045, 39.9189) knots 15 15 15 15 16 16 16 16
  line L865 (0.562, 39.9013) -> (0.5336, 39.898) construction
  line L866 (0.5336, 39.898) -> (0.5097, 39.9054) construction
  line L867 (0.5097, 39.9054) -> (0.5045, 39.9189) construction
  spline S162 degree 3 poles (3.2064, 39.9098) (3.1926, 39.9237) (3.1903, 42.3675) (3.2041, 42.3675) (3.2147, 42.3675) (3.3719, 42.246) (3.5362, 42.1108) knots 0 0 0 0 1 1 1 2 2 2 2
  line L868 (3.2064, 39.9098) -> (3.1926, 39.9237) construction
  line L869 (3.1926, 39.9237) -> (3.1903, 42.3675) construction
  line L870 (3.1903, 42.3675) -> (3.2041, 42.3675) construction
  line L871 (3.2041, 42.3675) -> (3.2147, 42.3675) construction
  line L872 (3.2147, 42.3675) -> (3.3719, 42.246) construction
  line L873 (3.3719, 42.246) -> (3.5362, 42.1108) construction
  spline S163 degree 3 poles (3.5362, 42.1108) (3.5957, 42.0618) (3.6761, 41.9983) (3.7148, 41.9697) (3.7534, 41.9411) (3.8734, 41.8463) (3.9814, 41.759) knots 2 2 2 2 3 3 3 4 4 4 4
  line L874 (3.5362, 42.1108) -> (3.5957, 42.0618) construction
  line L875 (3.5957, 42.0618) -> (3.6761, 41.9983) construction
  line L876 (3.6761, 41.9983) -> (3.7148, 41.9697) construction
  line L877 (3.7148, 41.9697) -> (3.7534, 41.9411) construction
  line L878 (3.7534, 41.9411) -> (3.8734, 41.8463) construction
  line L879 (3.8734, 41.8463) -> (3.9814, 41.759) construction
  spline S164 degree 3 poles (3.9814, 41.759) (4.4792, 41.3566) (4.4805, 41.3556) (4.5247, 41.3757) knots 4 4 4 4 5 5 5 5
  line L880 (3.9814, 41.759) -> (4.4792, 41.3566) construction
  line L881 (4.4792, 41.3566) -> (4.4805, 41.3556) construction
  line L882 (4.4805, 41.3556) -> (4.5247, 41.3757) construction
  spline S165 degree 3 poles (4.5247, 41.3757) (4.5472, 41.386) (4.6361, 41.4527) (4.7224, 41.5241) knots 5 5 5 5 6 6 6 6
  line L883 (4.5247, 41.3757) -> (4.5472, 41.386) construction
  line L884 (4.5472, 41.386) -> (4.6361, 41.4527) construction
  line L885 (4.6361, 41.4527) -> (4.7224, 41.5241) construction
  spline S166 degree 3 poles (4.7224, 41.5241) (4.8086, 41.5954) (4.9114, 41.6775) (4.9508, 41.7064) knots 6 6 6 6 7 7 7 7
  line L886 (4.7224, 41.5241) -> (4.8086, 41.5954) construction
  line L887 (4.8086, 41.5954) -> (4.9114, 41.6775) construction
  line L888 (4.9114, 41.6775) -> (4.9508, 41.7064) construction
  spline S167 degree 3 poles (4.9508, 41.7064) (4.9902, 41.7353) (5.0736, 41.8003) (5.136, 41.8508) knots 7 7 7 7 8 8 8 8
  line L889 (4.9508, 41.7064) -> (4.9902, 41.7353) construction
  line L890 (4.9902, 41.7353) -> (5.0736, 41.8003) construction
  line L891 (5.0736, 41.8003) -> (5.136, 41.8508) construction
  spline S168 degree 3 poles (5.136, 41.8508) (5.8001, 42.3875) (5.7853, 42.3764) (5.7967, 42.3465) knots 8 8 8 8 9 9 9 9
  line L892 (5.136, 41.8508) -> (5.8001, 42.3875) construction
  line L893 (5.8001, 42.3875) -> (5.7853, 42.3764) construction
  line L894 (5.7853, 42.3764) -> (5.7967, 42.3465) construction
  spline S169 degree 3 poles (5.7967, 42.3465) (5.8016, 42.3338) (5.8035, 41.7797) (5.801, 41.1151) knots 9 9 9 9 10 10 10 10
  line L895 (5.7967, 42.3465) -> (5.8016, 42.3338) construction
  line L896 (5.8016, 42.3338) -> (5.8035, 41.7797) construction
  line L897 (5.8035, 41.7797) -> (5.801, 41.1151) construction
  line L898 (5.801, 41.1151) -> (5.7964, 39.9069)
  line L899 (5.7964, 39.9069) -> (5.7347, 39.9069)
  line L900 (5.7347, 39.9069) -> (5.673, 39.9069)
  line L901 (5.673, 39.9069) -> (5.6641, 40.9948)
  line L902 (5.6641, 40.9948) -> (5.6553, 42.0827)
  line L903 (5.6553, 42.0827) -> (5.4659, 41.9296)
  spline S170 degree 3 poles (5.4659, 41.9296) (5.3618, 41.8455) (5.1845, 41.7052) (5.0721, 41.6179) (4.9596, 41.5305) (4.8027, 41.4068) (4.7235, 41.3429) knots 16 16 16 16 17 17 17 18 18 18 18
  line L904 (5.4659, 41.9296) -> (5.3618, 41.8455) construction
  line L905 (5.3618, 41.8455) -> (5.1845, 41.7052) construction
  line L906 (5.1845, 41.7052) -> (5.0721, 41.6179) construction
  line L907 (5.0721, 41.6179) -> (4.9596, 41.5305) construction
  line L908 (4.9596, 41.5305) -> (4.8027, 41.4068) construction
  line L909 (4.8027, 41.4068) -> (4.7235, 41.3429) construction
  spline S171 degree 3 poles (4.7235, 41.3429) (4.58, 41.2271) (4.5173, 41.1857) (4.4857, 41.1857) (4.4765, 41.1857) (4.4026, 41.2396) (4.3213, 41.3054) knots 18 18 18 18 19 19 19 20 20 20 20
  line L910 (4.7235, 41.3429) -> (4.58, 41.2271) construction
  line L911 (4.58, 41.2271) -> (4.5173, 41.1857) construction
  line L912 (4.5173, 41.1857) -> (4.4857, 41.1857) construction
  line L913 (4.4857, 41.1857) -> (4.4765, 41.1857) construction
  line L914 (4.4765, 41.1857) -> (4.4026, 41.2396) construction
  line L915 (4.4026, 41.2396) -> (4.3213, 41.3054) construction
  spline S172 degree 3 poles (4.3213, 41.3054) (4.2401, 41.3712) (4.1566, 41.4366) (4.1358, 41.4509) knots 20 20 20 20 21 21 21 21
  line L916 (4.3213, 41.3054) -> (4.2401, 41.3712) construction
  line L917 (4.2401, 41.3712) -> (4.1566, 41.4366) construction
  line L918 (4.1566, 41.4366) -> (4.1358, 41.4509) construction
  spline S173 degree 3 poles (4.1358, 41.4509) (4.1151, 41.4651) (4.0284, 41.5323) (3.9433, 41.6002) knots 21 21 21 21 22 22 22 22
  line L919 (4.1358, 41.4509) -> (4.1151, 41.4651) construction
  line L920 (4.1151, 41.4651) -> (4.0284, 41.5323) construction
  line L921 (4.0284, 41.5323) -> (3.9433, 41.6002) construction
  spline S174 degree 3 poles (3.9433, 41.6002) (3.329, 42.0903) (3.3441, 42.0795) (3.3288, 42.0397) knots 22 22 22 22 23 23 23 23
  line L922 (3.9433, 41.6002) -> (3.329, 42.0903) construction
  line L923 (3.329, 42.0903) -> (3.3441, 42.0795) construction
  line L924 (3.3441, 42.0795) -> (3.3288, 42.0397) construction
  spline S175 degree 3 poles (3.3288, 42.0397) (3.3232, 42.025) (3.3205, 41.5412) (3.3228, 40.9645) knots 23 23 23 23 24 24 24 24
  line L925 (3.3288, 42.0397) -> (3.3232, 42.025) construction
  line L926 (3.3232, 42.025) -> (3.3205, 41.5412) construction
  line L927 (3.3205, 41.5412) -> (3.3228, 40.9645) construction
  spline S176 degree 3 poles (3.3228, 40.9645) (3.3262, 40.1048) (3.3228, 39.9145) (3.3035, 39.9071) knots 24 24 24 24 25 25 25 25
  line L928 (3.3228, 40.9645) -> (3.3262, 40.1048) construction
  line L929 (3.3262, 40.1048) -> (3.3228, 39.9145) construction
  line L930 (3.3228, 39.9145) -> (3.3035, 39.9071) construction
  spline S177 degree 3 poles (3.3035, 39.9071) (3.2706, 39.8944) (3.2204, 39.8959) (3.2065, 39.9098) knots 25 25 25 25 26 26 26 26
  line L931 (3.3035, 39.9071) -> (3.2706, 39.8944) construction
  line L932 (3.2706, 39.8944) -> (3.2204, 39.8959) construction
  line L933 (3.2204, 39.8959) -> (3.2065, 39.9098) construction
  line L934 (3.2065, 39.9098) -> (3.2064, 39.9098)
  spline S178 degree 3 poles (0.7322, 41.0873) (0.7268, 41.1012) (0.7251, 41.131) (0.7283, 41.1536) knots 0 0 0 0 1 1 1 1
  line L935 (0.7322, 41.0873) -> (0.7268, 41.1012) construction
  line L936 (0.7268, 41.1012) -> (0.7251, 41.131) construction
  line L937 (0.7251, 41.131) -> (0.7283, 41.1536) construction
  line L938 (0.7283, 41.1536) -> (0.7341, 41.1945)
  line L939 (0.7341, 41.1945) -> (1.7748, 41.1945)
  line L940 (1.7748, 41.1945) -> (2.8154, 41.1945)
  line L941 (2.8154, 41.1945) -> (2.8154, 41.1328)
  line L942 (2.8154, 41.1328) -> (2.8154, 41.0711)
  line L943 (2.8154, 41.0711) -> (1.7787, 41.0665)
  spline S179 degree 3 poles (1.7787, 41.0665) (0.8912, 41.0626) (0.7405, 41.0656) (0.7322, 41.0873) knots 7 7 7 7 8 8 8 8
  line L944 (1.7787, 41.0665) -> (0.8912, 41.0626) construction
  line L945 (0.8912, 41.0626) -> (0.7405, 41.0656) construction
  line L946 (0.7405, 41.0656) -> (0.7322, 41.0873) construction
  spline S180 degree 3 poles (-7.553, 47.2226) (-7.5808, 47.2431) (-7.5827, 47.3337) (-7.5784, 48.4706) knots 0 0 0 0 1 1 1 1
  line L947 (-7.553, 47.2226) -> (-7.5808, 47.2431) construction
  line L948 (-7.5808, 47.2431) -> (-7.5827, 47.3337) construction
  line L949 (-7.5827, 47.3337) -> (-7.5784, 48.4706) construction
  line L950 (-7.5784, 48.4706) -> (-7.5739, 49.6965)
  line L951 (-7.5739, 49.6965) -> (-6.3138, 49.701)
  spline S181 degree 3 poles (-6.3138, 49.701) (-5.3174, 49.7046) (-5.0508, 49.7009) (-5.0396, 49.6834) knots 3 3 3 3 4 4 4 4
  line L952 (-6.3138, 49.701) -> (-5.3174, 49.7046) construction
  line L953 (-5.3174, 49.7046) -> (-5.0508, 49.7009) construction
  line L954 (-5.0508, 49.7009) -> (-5.0396, 49.6834) construction
  spline S182 degree 3 poles (-5.0396, 49.6834) (-5.0319, 49.6712) (-5.0255, 49.1165) (-5.0253, 48.4507) knots 4 4 4 4 5 5 5 5
  line L955 (-5.0396, 49.6834) -> (-5.0319, 49.6712) construction
  line L956 (-5.0319, 49.6712) -> (-5.0255, 49.1165) construction
  line L957 (-5.0255, 49.1165) -> (-5.0253, 48.4507) construction
  spline S183 degree 3 poles (-5.0253, 48.4507) (-5.025, 47.1195) (-5.0205, 47.1736) (-5.1275, 47.2112) knots 5 5 5 5 6 6 6 6
  line L958 (-5.0253, 48.4507) -> (-5.025, 47.1195) construction
  line L959 (-5.025, 47.1195) -> (-5.0205, 47.1736) construction
  line L960 (-5.0205, 47.1736) -> (-5.1275, 47.2112) construction
  line L961 (-5.1275, 47.2112) -> (-5.175, 47.2279)
  line L962 (-5.175, 47.2279) -> (-5.1795, 48.3872)
  line L963 (-5.1795, 48.3872) -> (-5.184, 49.5465)
  line L964 (-5.184, 49.5465) -> (-6.304, 49.5465)
  line L965 (-6.304, 49.5465) -> (-7.4239, 49.5465)
  line L966 (-7.4239, 49.5465) -> (-7.4239, 48.3843)
  spline S184 degree 3 poles (-7.4239, 48.3843) (-7.4239, 47.3407) (-7.4268, 47.2209) (-7.4518, 47.2113) knots 12 12 12 12 13 13 13 13
  line L967 (-7.4239, 48.3843) -> (-7.4239, 47.3407) construction
  line L968 (-7.4239, 47.3407) -> (-7.4268, 47.2209) construction
  line L969 (-7.4268, 47.2209) -> (-7.4518, 47.2113) construction
  spline S185 degree 3 poles (-7.4518, 47.2113) (-7.4936, 47.1952) (-7.5198, 47.1982) (-7.553, 47.2226) knots 13 13 13 13 14 14 14 14
  line L970 (-7.4518, 47.2113) -> (-7.4936, 47.1952) construction
  line L971 (-7.4936, 47.1952) -> (-7.5198, 47.1982) construction
  line L972 (-7.5198, 47.1982) -> (-7.553, 47.2226) construction
  spline S186 degree 3 poles (-12.7826, 47.2394) (-12.7987, 47.2554) (-12.8038, 47.5515) (-12.8038, 48.4638) (-12.8038, 49.1257) (-12.7989, 49.6797) (-12.7931, 49.695) knots 0 0 0 0 1 1 1 2 2 2 2
  line L973 (-12.7826, 47.2394) -> (-12.7987, 47.2554) construction
  line L974 (-12.7987, 47.2554) -> (-12.8038, 47.5515) construction
  line L975 (-12.8038, 47.5515) -> (-12.8038, 48.4638) construction
  line L976 (-12.8038, 48.4638) -> (-12.8038, 49.1257) construction
  line L977 (-12.8038, 49.1257) -> (-12.7989, 49.6797) construction
  line L978 (-12.7989, 49.6797) -> (-12.7931, 49.695) construction
  spline S187 degree 3 poles (-12.7931, 49.695) (-12.7834, 49.7201) (-12.6574, 49.7229) (-11.5495, 49.7229) knots 2 2 2 2 3 3 3 3
  line L979 (-12.7931, 49.695) -> (-12.7834, 49.7201) construction
  line L980 (-12.7834, 49.7201) -> (-12.6574, 49.7229) construction
  line L981 (-12.6574, 49.7229) -> (-11.5495, 49.7229) construction
  line L982 (-11.5495, 49.7229) -> (-10.3167, 49.7229)
  line L983 (-10.3167, 49.7229) -> (-10.3167, 49.6436)
  spline S188 degree 3 poles (-10.3167, 49.6436) (-10.3167, 49.5919) (-10.3244, 49.5641) (-10.3387, 49.5639) knots 5 5 5 5 6 6 6 6
  line L984 (-10.3167, 49.6436) -> (-10.3167, 49.5919) construction
  line L985 (-10.3167, 49.5919) -> (-10.3244, 49.5641) construction
  line L986 (-10.3244, 49.5641) -> (-10.3387, 49.5639) construction
  spline S189 degree 3 poles (-10.3387, 49.5639) (-10.3509, 49.5638) (-10.8708, 49.5639) (-11.4941, 49.5642) knots 6 6 6 6 7 7 7 7
  line L987 (-10.3387, 49.5639) -> (-10.3509, 49.5638) construction
  line L988 (-10.3509, 49.5638) -> (-10.8708, 49.5639) construction
  line L989 (-10.8708, 49.5639) -> (-11.4941, 49.5642) construction
  line L990 (-11.4941, 49.5642) -> (-12.6274, 49.5647)
  line L991 (-12.6274, 49.5647) -> (-12.6274, 48.4796)
  line L992 (-12.6274, 48.4796) -> (-12.6274, 47.3946)
  line L993 (-12.6274, 47.3946) -> (-11.4999, 47.3946)
  spline S190 degree 3 poles (-11.4999, 47.3946) (-10.8798, 47.3946) (-10.3599, 47.3898) (-10.3446, 47.3839) knots 11 11 11 11 12 12 12 12
  line L994 (-11.4999, 47.3946) -> (-10.8798, 47.3946) construction
  line L995 (-10.8798, 47.3946) -> (-10.3599, 47.3898) construction
  line L996 (-10.3599, 47.3898) -> (-10.3446, 47.3839) construction
  spline S191 degree 3 poles (-10.3446, 47.3839) (-10.3061, 47.3691) (-10.3061, 47.2437) (-10.3446, 47.2289) knots 12 12 12 12 13 13 13 13
  line L997 (-10.3446, 47.3839) -> (-10.3061, 47.3691) construction
  line L998 (-10.3061, 47.3691) -> (-10.3061, 47.2437) construction
  line L999 (-10.3061, 47.2437) -> (-10.3446, 47.2289) construction
  spline S192 degree 3 poles (-10.3446, 47.2289) (-10.3599, 47.223) (-10.91, 47.2182) (-11.567, 47.2182) (-12.4725, 47.2182) (-12.7666, 47.2233) (-12.7826, 47.2394) knots 13 13 13 13 14 14 14 15 15 15 15
  line L1000 (-10.3446, 47.2289) -> (-10.3599, 47.223) construction
  line L1001 (-10.3599, 47.223) -> (-10.91, 47.2182) construction
  line L1002 (-10.91, 47.2182) -> (-11.567, 47.2182) construction
  line L1003 (-11.567, 47.2182) -> (-12.4725, 47.2182) construction
  line L1004 (-12.4725, 47.2182) -> (-12.7666, 47.2233) construction
  line L1005 (-12.7666, 47.2233) -> (-12.7826, 47.2394) construction
  spline S193 degree 3 poles (-10.1359, 47.2299) (-10.1532, 47.2369) (-10.1579, 47.5039) (-10.1579, 48.4819) knots 0 0 0 0 1 1 1 1
  line L1006 (-10.1359, 47.2299) -> (-10.1532, 47.2369) construction
  line L1007 (-10.1532, 47.2369) -> (-10.1579, 47.5039) construction
  line L1008 (-10.1579, 47.5039) -> (-10.1579, 48.4819) construction
  line L1009 (-10.1579, 48.4819) -> (-10.1579, 49.725)
  line L1010 (-10.1579, 49.725) -> (-10.083, 49.7195)
  line L1011 (-10.083, 49.7195) -> (-10.008, 49.7141)
  line L1012 (-10.008, 49.7141) -> (-10.0034, 49.1364)
  line L1013 (-10.0034, 49.1364) -> (-9.9987, 48.5588)
  line L1014 (-9.9987, 48.5588) -> (-8.932, 48.5588)
  line L1015 (-8.932, 48.5588) -> (-7.8654, 48.5588)
  line L1016 (-7.8654, 48.5588) -> (-7.8607, 49.1364)
  line L1017 (-7.8607, 49.1364) -> (-7.8561, 49.7141)
  line L1018 (-7.8561, 49.7141) -> (-7.7811, 49.7195)
  line L1019 (-7.7811, 49.7195) -> (-7.7062, 49.725)
  line L1020 (-7.7062, 49.725) -> (-7.7062, 48.4807)
  line L1021 (-7.7062, 48.4807) -> (-7.7062, 47.2365)
  line L1022 (-7.7062, 47.2365) -> (-7.749, 47.2258)
  spline S194 degree 3 poles (-7.749, 47.2258) (-7.7725, 47.2199) (-7.8082, 47.2203) (-7.8283, 47.2266) knots 15 15 15 15 16 16 16 16
  line L1023 (-7.749, 47.2258) -> (-7.7725, 47.2199) construction
  line L1024 (-7.7725, 47.2199) -> (-7.8082, 47.2203) construction
  line L1025 (-7.8082, 47.2203) -> (-7.8283, 47.2266) construction
  spline S195 degree 3 poles (-7.8283, 47.2266) (-7.8643, 47.238) (-7.8649, 47.2471) (-7.8649, 47.8103) knots 16 16 16 16 17 17 17 17
  line L1026 (-7.8283, 47.2266) -> (-7.8643, 47.238) construction
  line L1027 (-7.8643, 47.238) -> (-7.8649, 47.2471) construction
  line L1028 (-7.8649, 47.2471) -> (-7.8649, 47.8103) construction
  line L1029 (-7.8649, 47.8103) -> (-7.8649, 48.3824)
  line L1030 (-7.8649, 48.3824) -> (-8.932, 48.3824)
  line L1031 (-8.932, 48.3824) -> (-9.9992, 48.3824)
  line L1032 (-9.9992, 48.3824) -> (-9.9992, 47.811)
  spline S196 degree 3 poles (-9.9992, 47.811) (-9.9992, 47.3062) (-10.0024, 47.2384) (-10.0271, 47.2289) knots 21 21 21 21 22 22 22 22
  line L1033 (-9.9992, 47.811) -> (-9.9992, 47.3062) construction
  line L1034 (-9.9992, 47.3062) -> (-10.0024, 47.2384) construction
  line L1035 (-10.0024, 47.2384) -> (-10.0271, 47.2289) construction
  spline S197 degree 3 poles (-10.0271, 47.2289) (-10.0592, 47.2166) (-10.104, 47.217) (-10.1359, 47.2299) knots 22 22 22 22 23 23 23 23
  line L1036 (-10.0271, 47.2289) -> (-10.0592, 47.2166) construction
  line L1037 (-10.0592, 47.2166) -> (-10.104, 47.217) construction
  line L1038 (-10.104, 47.217) -> (-10.1359, 47.2299) construction